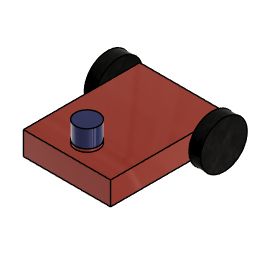
lidar v1 (Autodesk Fusion 360 design; units mm, degrees)
Autodesk Fusion 360 part; units mm, degrees
sketch "Sketch1" plane through (0, 0, 0) normal (0, 0, 1) x (1, 0, 0)
  line L0 (75, -100) -> (-75, -100)
  line L1 (-75, -100) -> (-75, 100)
  line L2 (-75, 100) -> (75, 100)
  line L3 (75, 100) -> (75, -100)
  line L4 (75, -100) -> (-75, 100) construction
  line L5 (-75, -100) -> (75, 100) construction
  dimension "d1" = 200
  dimension "d2" = 150
  constraint horizontal L0
  constraint perpendicular L0 L1
  constraint parallel L0 L2
  constraint parallel L1 L3
  constraint coincident L4 origin
  constraint coincident L5 origin
  measures "d1" distance of L0.end L1.end
  measures "d2" distance of L1.end L2.end
extrude "Extrude1" add sketch "Sketch1" along normal blind 40 makes body 1
sketch "Sketch2" plane through (75, 0, 0) normal (1, 0, 0) x (0, 1, 0)
  line L0 (-100, 0) -> (100, 0)
  line L1 (100, 0) -> (100, 40)
  line L2 (100, 40) -> (-100, 40)
  line L3 (-100, 40) -> (-100, 0)
  circle A0 centre (70, 20) radius 5
  dimension "d5" = 10
  measures "d5" diameter of A0
sketch "Sketch3" plane through (-75, 0, 0) normal (-1, 0, 0) x (0, -1, 0)
  line L0 (-100, 0) -> (100, 0)
  line L1 (100, 0) -> (100, 40)
  line L2 (100, 40) -> (-100, 40)
  line L3 (-100, 40) -> (-100, 0)
  circle A0 centre (-70, 20) radius 5
  dimension "d6" = 10
  measures "d6" diameter of A0
extrude "Extrude2" add sketch "Sketch2" along normal blind 5 contours A0 bodies 1
extrude "Extrude3" add sketch "Sketch3" along normal blind 5 contours A0 bodies 1
sketch "Sketch4" plane through (80, 0, 0) normal (1, 0, 0) x (0, 1, 0)
  circle A0 centre (70, 20) radius 5
sketch "Sketch5" plane through (80, 0, 0) normal (1, 0, 0) x (0, 1, 0)
  circle A0 centre (70, 20) radius 40
  dimension "d11" = 80
  measures "d11" diameter of A0
extrude "Extrude4" add sketch "Sketch5" sketch "Sketch4" along normal blind 20 separate body of sketch 2 makes body 2
sketch "Sketch6" plane through (-80, 0, 0) normal (-1, 0, 0) x (0, -1, 0)
  circle A0 centre (-70, 20) radius 5
  circle A1 centre (-70, 20) radius 40
  dimension "d14" = 80
  constraint concentric A0 A1
  measures "d14" diameter of A1
extrude "Extrude5" add sketch "Sketch6" along normal blind 20 separate body contours A0 | A1 makes body 3
sketch "Sketch7" plane through (0, 0, 0) normal (0, 0, -1) x (1, 0, 0)
  line L0 (-75, -100) -> (75, -100)
  line L1 (75, -100) -> (75, 100)
  line L2 (75, 100) -> (-75, 100)
  line L3 (-75, 100) -> (-75, -100)
  circle A0 centre (0, 70) radius 10
  dimension "d17" = 20
  measures "d17" diameter of A0
extrude "Extrude6" add sketch "Sketch7" along normal blind 20 contours A0 bodies 1
fillet "Fillet1" radius 10 1 faces at (3.0744, -69.5032, -20) on bodies 1
sketch "Sketch8" plane through (0, 0, 40) normal (0, 0, 1) x (-1, 0, 0)
  line L0 (-75, -100) -> (75, -100)
  line L1 (75, -100) -> (75, 100)
  line L2 (75, 100) -> (-75, 100)
  line L3 (-75, 100) -> (-75, -100)
  circle A0 centre (0.6581, 64.8262) radius 20
  dimension "d22" = 40
  measures "d22" diameter of A0
extrude "Extrude7" add sketch "Sketch8" along normal blind 5 contours A0 bodies 1
extrude "Extrude8" add 1 faces at (-8.4731, -58.1782, 45) along direction (0, 0, 1) blind 30 separate body on bodies 1 makes body 4
copy_body "Body->Comp1" bodies 1 removing the originals makes body 5 in component "old_component"
copy_body "Body->Comp2" bodies 2 removing the originals makes body 6 in component "old_component (1)"
copy_body "Body->Comp3" bodies 3 removing the originals makes body 7 in component "old_component (2)"
copy_body "Body->Comp4" bodies 4 removing the originals makes body 8 in component "old_component (3)"
copy_body "CopyPasteBodies1" bodies 5 makes body 9 in component "base_link"
copy_body "CopyPasteBodies1'" bodies 6 makes body 10 in component "left_wheel_1"
copy_body "CopyPasteBodies1''" bodies 7 makes body 11 in component "right_wheel_1"
copy_body "CopyPasteBodies1'''" bodies 8 makes body 12 in component "lidar_1"
component "old_component" placed x (1, 0, 0) y (0, 1, 0) z (0, 0, 1) at (0, 0, 0)
component "old_component (1)" placed x (1, 0, 0) y (0, 1, 0) z (0, 0, 1) at (0, 0, 0)
component "old_component (2)" placed x (1, 0, 0) y (0, 1, 0) z (0, 0, 1) at (0, 0, 0)
component "old_component (3)" placed x (1, 0, 0) y (0, 1, 0) z (0, 0, 1) at (0, 0, 0)
component "base_link" placed x (1, 0, 0) y (0, 1, 0) z (0, 0, 1) at (0, 0, 0)
component "left_wheel_1" placed x (1, 0, 0) y (0, 1, 0) z (0, 0, 1) at (0, 0, 0)
component "right_wheel_1" placed x (1, 0, 0) y (0, 1, 0) z (0, 0, 1) at (0, 0, 0)
component "lidar_1" placed x (1, 0, 0) y (0, 1, 0) z (0, 0, 1) at (0, 0, 0)
named bodies: "base_link", "left_wheel", "right_wheel", "lidar"
